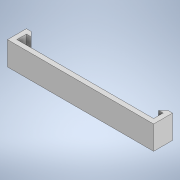
# Autodesk Inventor part: Крышка аккумулятора
Saved by Autodesk Inventor 2020 (Build 240168000, 168)
## iProperties
Created: 2021-04-26
Part Number: Крышка аккумулятора
Material: Типовые
Document SubType Name: Modeling
Designer: Антон
Density: 1 g/cm^3
Appearance: По умолчанию
Author: Антон
Autodesk Inventor part; units mm, degrees
ref_plane "YZ Plane" through (0, 0, 0) normal (1, 0, 0) x (0, 1, 0)
ref_plane "XZ Plane" through (0, 0, 0) normal (0, 1, 0) x (-1, 0, 0)
ref_plane "XY Plane" through (0, 0, 0) normal (0, 0, 1) x (1, 0, 0)
sketch "Эскиз1" plane through (0, 0, 0) normal (0, 0, 1) x (1, 0, 0)
  line L0 (0, 0) -> (61.8, 0)
  line L1 (61.8, 0) -> (61.8, 10)
  line L2 (61.8, 10) -> (0, 10)
  line L3 (0, 10) -> (0, 0)
  dimension "d0" = 61.8
  dimension "d1" = 10
  constraints: 8 end point, 2 parallel, 1 horizontal, 1 perpendicular
  measures "d0" distance of L2.end L1.end
  measures "d1" distance of L1.end L0.end
extrude "Выдавливание1" add sketch "Эскиз1" along normal blind 2
sketch "Эскиз2" plane through (0, 10, 0) normal (0, 1, 0) x (1, 0, 0)
  line L0 (0, 0) -> (2, 0)
  line L1 (2, 0) -> (2, 6)
  line L2 (2, 6) -> (0, 6)
  line L3 (0, 6) -> (0, 0)
  line L4 (2, 6) -> (4, 6)
  line L5 (4, 6) -> (4, 4)
  line L6 (4, 4) -> (2, 4)
  line L7 (2, 4) -> (2, 6)
  line L8 (4, 4) -> (2, 6)
  dimension "d4" = 2
  dimension "d5" = 6
  dimension "d6" = 2
  dimension "d7" = 2
  constraints: 18 end point, 4 parallel, 2 horizontal, 2 perpendicular
  measures "d4" distance of L2.end L1.end
  measures "d5" distance of L1.end L0.end
  measures "d6" distance of L5.end L6.end
  measures "d7" distance of L4.end L5.end
extrude "Выдавливание2" add sketch "Эскиз2" against normal up to surface (10 mm away) contours L3 L2 L1 L0 | L1 L8 L6
ref_plane "РабПлоскость1" through (30.9, 0, 2) normal (-1, 0, 0) x (0, 0, 1)
mirror "Зеркальное отражение1" about plane through (30.9, 0, 2) normal (-1, 0, 0) of "Выдавливание2"
